Autodesk Fusion 360 part; units mm, degrees
(part 2 of 6)
  spline S17 degree 5 poles (103.1872, 58.6334) (103.1759, 58.6333) (103.1533, 58.6329) (103.1196, 58.6324) (103.0746, 58.6315) (103.0184, 58.6301) (102.9623, 58.6285) (102.9063, 58.6266) (102.8503, 58.6245) (102.7945, 58.6221) (102.7387, 58.6195) (102.683, 58.6167) (102.6274, 58.6136) (102.5718, 58.6103) (102.5164, 58.6067) (102.461, 58.6029) (102.4058, 58.5988) (102.3506, 58.5945) (102.2955, 58.5899) (102.2405, 58.585) (102.1856, 58.5799) (102.1308, 58.5746) (102.0761, 58.5689) (102.0215, 58.5631) (101.967, 58.5569) (101.9126, 58.5505) (101.8583, 58.5438) (101.8041, 58.5369) (101.75, 58.5297) (101.6961, 58.5222) (101.6422, 58.5144) (101.5884, 58.5064) (101.5348, 58.4981) (101.4813, 58.4895) (101.4279, 58.4806) (101.3746, 58.4714) (101.3215, 58.462) (101.2685, 58.4522) (101.2156, 58.4422) (101.1628, 58.4319) (101.1102, 58.4212) (101.0577, 58.4103) (101.0053, 58.3991) (100.9531, 58.3875) (100.9011, 58.3756) (100.8492, 58.3634) (100.7974, 58.3509) (100.7458, 58.3381) (100.6943, 58.325) (100.643, 58.3115) (100.5919, 58.2977) (100.541, 58.2835) (100.4902, 58.2689) (100.4397, 58.254) (100.3893, 58.2386) (100.3392, 58.223) (100.2892, 58.2069) (100.2393, 58.1906) (100.1897, 58.1739) (100.1403, 58.1567) (100.0911, 58.1391) (100.0423, 58.1209) (99.9938, 58.1022) (99.9456, 58.0828) (99.8977, 58.0629) (99.85, 58.0426) (99.8025, 58.022) (99.7552, 58.0012) (99.7081, 57.9799) (99.6615, 57.9579) (99.6156, 57.9346) (99.5797, 57.9146) (99.5534, 57.8987) (99.536, 57.8877) (99.5274, 57.882) knots -1 -1 -1 -1 -1 -1 -0.98571429 -0.97142857 -0.95714286 -0.94285714 -0.92857143 -0.91428571 -0.9 -0.88571429 -0.87142857 -0.85714286 -0.84285714 -0.82857143 -0.81428571 -0.8 -0.78571429 -0.77142857 -0.75714286 -0.74285714 -0.72857143 -0.71428571 -0.7 -0.68571429 -0.67142857 -0.65714286 -0.64285714 -0.62857143 -0.61428571 -0.6 -0.58571429 -0.57142857 -0.55714286 -0.54285714 -0.52857143 -0.51428571 -0.5 -0.48571429 -0.47142857 -0.45714286 -0.44285714 -0.42857143 -0.41428571 -0.4 -0.38571429 -0.37142857 -0.35714286 -0.34285714 -0.32857143 -0.31428571 -0.3 -0.28571429 -0.27142857 -0.25714286 -0.24285714 -0.22857143 -0.21428571 -0.2 -0.18571429 -0.17142857 -0.15714286 -0.14285714 -0.12857143 -0.11428571 -0.1 -0.08571429 -0.07142857 -0.05714286 -0.04285714 -0.02857143 -0.01428571 0 0 0 0 0 0
  line L17 (99.5274, 57.882) -> (99.1106, 57.6092)
  arc A35 (98.4247, 57.7443) -> (99.1106, 57.6092) centre (98.8368, 58.0275) ccw
  arc A36 (98.4247, 57.7443) -> (97.7326, 58.697) centre (79.882, 45) ccw
  arc A37 (97.816, 59.3911) -> (97.7326, 58.697) centre (98.1293, 59.0013) ccw
  line L18 (97.816, 59.3911) -> (98.2043, 59.7031)
  spline S18 degree 5 poles (98.2043, 59.7031) (98.2123, 59.7096) (98.2282, 59.7226) (98.2515, 59.7428) (98.2816, 59.7708) (98.3179, 59.8072) (98.3533, 59.8447) (98.388, 59.8829) (98.4225, 59.9215) (98.4567, 59.9603) (98.4907, 59.9994) (98.5245, 60.0388) (98.5578, 60.0786) (98.5906, 60.1189) (98.623, 60.1598) (98.655, 60.2011) (98.6865, 60.2428) (98.7177, 60.2848) (98.7487, 60.3272) (98.7794, 60.3698) (98.8098, 60.4127) (98.84, 60.4558) (98.8698, 60.4993) (98.8993, 60.543) (98.9286, 60.5871) (98.9575, 60.6314) (98.9862, 60.676) (99.0146, 60.7209) (99.0427, 60.766) (99.0706, 60.8114) (99.0982, 60.857) (99.1256, 60.9028) (99.1527, 60.9489) (99.1796, 60.9952) (99.2062, 61.0418) (99.2326, 61.0885) (99.2587, 61.1355) (99.2846, 61.1827) (99.3103, 61.2302) (99.3357, 61.2778) (99.3609, 61.3256) (99.3858, 61.3737) (99.4105, 61.4219) (99.435, 61.4703) (99.4593, 61.519) (99.4833, 61.5678) (99.5071, 61.6168) (99.5307, 61.666) (99.554, 61.7154) (99.5771, 61.765) (99.6, 61.8148) (99.6227, 61.8647) (99.6452, 61.9148) (99.6674, 61.9651) (99.6895, 62.0156) (99.7113, 62.0662) (99.7329, 62.117) (99.7543, 62.168) (99.7755, 62.2191) (99.7964, 62.2704) (99.8172, 62.3219) (99.8377, 62.3735) (99.858, 62.4253) (99.8782, 62.4772) (99.8981, 62.5293) (99.9178, 62.5816) (99.9373, 62.634) (99.9566, 62.6865) (99.9756, 62.7392) (99.9945, 62.7921) (100.0132, 62.8451) (100.028, 62.8876) (100.039, 62.9195) (100.0462, 62.9409) (100.0499, 62.9515) knots 0 0 0 0 0 0 0.01428571 0.02857143 0.04285714 0.05714286 0.07142857 0.08571429 0.1 0.11428571 0.12857143 0.14285714 0.15714286 0.17142857 0.18571429 0.2 0.21428571 0.22857143 0.24285714 0.25714286 0.27142857 0.28571429 0.3 0.31428571 0.32857143 0.34285714 0.35714286 0.37142857 0.38571429 0.4 0.41428571 0.42857143 0.44285714 0.45714286 0.47142857 0.48571429 0.5 0.51428571 0.52857143 0.54285714 0.55714286 0.57142857 0.58571429 0.6 0.61428571 0.62857143 0.64285714 0.65714286 0.67142857 0.68571429 0.7 0.71428571 0.72857143 0.74285714 0.75714286 0.77142857 0.78571429 0.8 0.81428571 0.82857143 0.84285714 0.85714286 0.87142857 0.88571429 0.9 0.91428571 0.92857143 0.94285714 0.95714286 0.97142857 0.98571429 1 1 1 1 1 1
  arc A38 (100.0499, 62.9515) -> (99.0645, 64.0009) centre (79.882, 45) ccw
  spline S19 degree 5 poles (99.0645, 64.0009) (99.0536, 63.9979) (99.0319, 63.992) (98.9993, 63.983) (98.9559, 63.9709) (98.9019, 63.9556) (98.8479, 63.9401) (98.7941, 63.9244) (98.7405, 63.9084) (98.687, 63.8923) (98.6336, 63.8759) (98.5803, 63.8593) (98.5272, 63.8425) (98.4743, 63.8254) (98.4215, 63.8082) (98.3688, 63.7907) (98.3163, 63.773) (98.2639, 63.7551) (98.2117, 63.7369) (98.1596, 63.7186) (98.1077, 63.7) (98.056, 63.6811) (98.0044, 63.6621) (97.953, 63.6428) (97.9017, 63.6233) (97.8506, 63.6036) (97.7997, 63.5836) (97.7489, 63.5634) (97.6983, 63.543) (97.6479, 63.5223) (97.5977, 63.5014) (97.5476, 63.4802) (97.4977, 63.4588) (97.448, 63.4372) (97.3985, 63.4153) (97.3492, 63.3932) (97.3001, 63.3708) (97.2511, 63.3482) (97.2024, 63.3253) (97.1538, 63.3022) (97.1055, 63.2788) (97.0574, 63.2552) (97.0095, 63.2313) (96.9618, 63.2071) (96.9143, 63.1826) (96.8671, 63.1579) (96.8201, 63.1329) (96.7733, 63.1077) (96.7267, 63.0822) (96.6803, 63.0564) (96.6343, 63.0303) (96.5885, 63.0038) (96.5429, 62.9771) (96.4977, 62.9501) (96.4527, 62.9227) (96.408, 62.895) (96.3636, 62.8671) (96.3194, 62.8388) (96.2755, 62.8103) (96.2319, 62.7814) (96.1886, 62.7521) (96.1458, 62.7224) (96.1035, 62.6921) (96.0617, 62.6614) (96.0202, 62.6302) (95.9791, 62.5987) (95.9382, 62.567) (95.8976, 62.535) (95.8573, 62.5027) (95.8176, 62.4697) (95.779, 62.4358) (95.7492, 62.4075) (95.7276, 62.3855) (95.7135, 62.3705) (95.7066, 62.3629) knots -1 -1 -1 -1 -1 -1 -0.98571429 -0.97142857 -0.95714286 -0.94285714 -0.92857143 -0.91428571 -0.9 -0.88571429 -0.87142857 -0.85714286 -0.84285714 -0.82857143 -0.81428571 -0.8 -0.78571429 -0.77142857 -0.75714286 -0.74285714 -0.72857143 -0.71428571 -0.7 -0.68571429 -0.67142857 -0.65714286 -0.64285714 -0.62857143 -0.61428571 -0.6 -0.58571429 -0.57142857 -0.55714286 -0.54285714 -0.52857143 -0.51428571 -0.5 -0.48571429 -0.47142857 -0.45714286 -0.44285714 -0.42857143 -0.41428571 -0.4 -0.38571429 -0.37142857 -0.35714286 -0.34285714 -0.32857143 -0.31428571 -0.3 -0.28571429 -0.27142857 -0.25714286 -0.24285714 -0.22857143 -0.21428571 -0.2 -0.18571429 -0.17142857 -0.15714286 -0.14285714 -0.12857143 -0.11428571 -0.1 -0.08571429 -0.07142857 -0.05714286 -0.04285714 -0.02857143 -0.01428571 0 0 0 0 0 0
  line L19 (95.7066, 62.3629) -> (95.3708, 61.995)
  arc A39 (94.6728, 61.9553) -> (95.3708, 61.995) centre (95.0015, 62.3321) ccw
  arc A40 (94.6728, 61.9553) -> (93.7655, 62.7059) centre (79.882, 45) ccw
  arc A41 (93.6737, 63.3989) -> (93.7655, 62.7059) centre (94.074, 63.0994) ccw
  line L20 (93.6737, 63.3989) -> (93.9722, 63.7978)
  spline S20 degree 5 poles (93.9722, 63.7978) (93.9783, 63.806) (93.9905, 63.8226) (94.008, 63.8479) (94.0302, 63.8825) (94.0563, 63.9268) (94.0812, 63.972) (94.1054, 64.0176) (94.1292, 64.0635) (94.1527, 64.1096) (94.1759, 64.1559) (94.1988, 64.2025) (94.2212, 64.2494) (94.2429, 64.2966) (94.2642, 64.3442) (94.2848, 64.3922) (94.305, 64.4404) (94.3248, 64.4889) (94.3443, 64.5376) (94.3634, 64.5865) (94.3822, 64.6356) (94.4007, 64.6849) (94.4188, 64.7344) (94.4365, 64.7841) (94.4539, 64.8341) (94.4709, 64.8842) (94.4875, 64.9346) (94.5039, 64.9851) (94.5199, 65.0358) (94.5356, 65.0867) (94.5511, 65.1377) (94.5662, 65.1889) (94.581, 65.2403) (94.5955, 65.2918) (94.6097, 65.3435) (94.6236, 65.3954) (94.6372, 65.4474) (94.6506, 65.4996) (94.6636, 65.5519) (94.6764, 65.6043) (94.6889, 65.6569) (94.7011, 65.7096) (94.713, 65.7625) (94.7247, 65.8155) (94.7361, 65.8687) (94.7472, 65.9219) (94.7581, 65.9753) (94.7687, 66.0289) (94.779, 66.0825) (94.7891, 66.1363) (94.7989, 66.1902) (94.8085, 66.2442) (94.8178, 66.2983) (94.8268, 66.3525) (94.8356, 66.4069) (94.8441, 66.4614) (94.8524, 66.516) (94.8605, 66.5706) (94.8683, 66.6254) (94.8758, 66.6803) (94.8831, 66.7354) (94.8902, 66.7905) (94.897, 66.8457) (94.9035, 66.901) (94.9099, 66.9564) (94.916, 67.0119) (94.9218, 67.0675) (94.9274, 67.1232) (94.9328, 67.179) (94.9379, 67.2349) (94.9428, 67.2909) (94.9466, 67.3357) (94.9493, 67.3694) (94.951, 67.3919) (94.9519, 67.4031) knots 0 0 0 0 0 0 0.01428571 0.02857143 0.04285714 0.05714286 0.07142857 0.08571429 0.1 0.11428571 0.12857143 0.14285714 0.15714286 0.17142857 0.18571429 0.2 0.21428571 0.22857143 0.24285714 0.25714286 0.27142857 0.28571429 0.3 0.31428571 0.32857143 0.34285714 0.35714286 0.37142857 0.38571429 0.4 0.41428571 0.42857143 0.44285714 0.45714286 0.47142857 0.48571429 0.5 0.51428571 0.52857143 0.54285714 0.55714286 0.57142857 0.58571429 0.6 0.61428571 0.62857143 0.64285714 0.65714286 0.67142857 0.68571429 0.7 0.71428571 0.72857143 0.74285714 0.75714286 0.77142857 0.78571429 0.8 0.81428571 0.82857143 0.84285714 0.85714286 0.87142857 0.88571429 0.9 0.91428571 0.92857143 0.94285714 0.95714286 0.97142857 0.98571429 1 1 1 1 1 1
  arc A42 (94.9519, 67.4031) -> (93.7365, 68.1744) centre (79.882, 45) ccw
  spline S21 degree 5 poles (93.7365, 68.1744) (93.7267, 68.1688) (93.7071, 68.1577) (93.6778, 68.1409) (93.6388, 68.1184) (93.5902, 68.0902) (93.5419, 68.0617) (93.4937, 68.0331) (93.4457, 68.0043) (93.3978, 67.9753) (93.3502, 67.9462) (93.3028, 67.9169) (93.2555, 67.8874) (93.2085, 67.8577) (93.1616, 67.8278) (93.1149, 67.7978) (93.0685, 67.7676) (93.0222, 67.7372) (92.9761, 67.7067) (92.9303, 67.6759) (92.8846, 67.645) (92.8392, 67.6139) (92.794, 67.5826) (92.749, 67.5512) (92.7042, 67.5195) (92.6596, 67.4877) (92.6152, 67.4557) (92.5711, 67.4235) (92.5271, 67.3911) (92.4834, 67.3586) (92.44, 67.3258) (92.3968, 67.2929) (92.3538, 67.2598) (92.311, 67.2264) (92.2685, 67.1929) (92.2262, 67.1592) (92.1842, 67.1254) (92.1424, 67.0913) (92.1009, 67.057) (92.0596, 67.0225) (92.0186, 66.9879) (91.9779, 66.953) (91.9375, 66.9179) (91.8973, 66.8826) (91.8574, 66.8472) (91.8178, 66.8115) (91.7784, 66.7756) (91.7394, 66.7395) (91.7006, 66.7032) (91.6622, 66.6667) (91.624, 66.6299) (91.5862, 66.5929) (91.5488, 66.5557) (91.5117, 66.5183) (91.4749, 66.4806) (91.4385, 66.4427) (91.4024, 66.4045) (91.3667, 66.3662) (91.3312, 66.3276) (91.2961, 66.2888) (91.2616, 66.2497) (91.2275, 66.2102) (91.194, 66.1704) (91.1612, 66.1302) (91.1288, 66.0897) (91.0968, 66.049) (91.0651, 66.0081) (91.0336, 65.967) (91.0027, 65.9257) (90.9724, 65.8839) (90.9434, 65.8414) (90.9216, 65.8066) (90.9061, 65.78) (90.8963, 65.7619) (90.8915, 65.7529) knots -1 -1 -1 -1 -1 -1 -0.98571429 -0.97142857 -0.95714286 -0.94285714 -0.92857143 -0.91428571 -0.9 -0.88571429 -0.87142857 -0.85714286 -0.84285714 -0.82857143 -0.81428571 -0.8 -0.78571429 -0.77142857 -0.75714286 -0.74285714 -0.72857143 -0.71428571 -0.7 -0.68571429 -0.67142857 -0.65714286 -0.64285714 -0.62857143 -0.61428571 -0.6 -0.58571429 -0.57142857 -0.55714286 -0.54285714 -0.52857143 -0.51428571 -0.5 -0.48571429 -0.47142857 -0.45714286 -0.44285714 -0.42857143 -0.41428571 -0.4 -0.38571429 -0.37142857 -0.35714286 -0.34285714 -0.32857143 -0.31428571 -0.3 -0.28571429 -0.27142857 -0.25714286 -0.24285714 -0.22857143 -0.21428571 -0.2 -0.18571429 -0.17142857 -0.15714286 -0.14285714 -0.12857143 -0.11428571 -0.1 -0.08571429 -0.07142857 -0.05714286 -0.04285714 -0.02857143 -0.01428571 0 0 0 0 0 0
  line L21 (90.8915, 65.7529) -> (90.6577, 65.313)
  arc A43 (89.9915, 65.101) -> (90.6577, 65.313) centre (90.2161, 65.5476) ccw
  arc A44 (89.9915, 65.101) -> (88.926, 65.6023) centre (79.882, 45) ccw
  arc A45 (88.6648, 66.2508) -> (88.926, 65.6023) centre (89.127, 66.0601) ccw
  line L22 (88.6648, 66.2508) -> (88.8547, 66.7113)
  spline S22 degree 5 poles (88.8547, 66.7113) (88.8586, 66.7208) (88.8662, 66.7399) (88.8769, 66.7688) (88.8898, 66.8078) (88.9041, 66.8572) (88.917, 66.9071) (88.929, 66.9573) (88.9407, 67.0077) (88.952, 67.0582) (88.963, 67.1089) (88.9735, 67.1596) (88.9835, 67.2106) (88.9929, 67.2618) (89.0016, 67.3132) (89.0097, 67.3647) (89.0173, 67.4165) (89.0244, 67.4684) (89.0311, 67.5204) (89.0375, 67.5725) (89.0435, 67.6247) (89.0491, 67.6771) (89.0543, 67.7295) (89.0591, 67.7821) (89.0635, 67.8348) (89.0675, 67.8876) (89.0711, 67.9405) (89.0744, 67.9935) (89.0773, 68.0466) (89.0799, 68.0998) (89.0822, 68.1531) (89.0841, 68.2064) (89.0856, 68.2599) (89.0869, 68.3134) (89.0878, 68.367) (89.0884, 68.4207) (89.0886, 68.4745) (89.0886, 68.5283) (89.0882, 68.5822) (89.0875, 68.6362) (89.0865, 68.6903) (89.0852, 68.7444) (89.0837, 68.7985) (89.0818, 68.8528) (89.0796, 68.9071) (89.0771, 68.9615) (89.0744, 69.0159) (89.0713, 69.0704) (89.068, 69.1249) (89.0644, 69.1795) (89.0605, 69.2341) (89.0563, 69.2888) (89.0518, 69.3435) (89.0471, 69.3983) (89.0421, 69.4532) (89.0368, 69.5081) (89.0313, 69.563) (89.0255, 69.618) (89.0194, 69.673) (89.0131, 69.728) (89.0064, 69.7831) (88.9996, 69.8382) (88.9924, 69.8934) (88.9851, 69.9486) (88.9774, 70.0039) (88.9695, 70.0592) (88.9613, 70.1145) (88.9529, 70.1698) (88.9443, 70.2252) (88.9353, 70.2806) (88.9262, 70.336) (88.9186, 70.3804) (88.9129, 70.4137) (88.909, 70.4359) (88.907, 70.447) knots 0 0 0 0 0 0 0.01428571 0.02857143 0.04285714 0.05714286 0.07142857 0.08571429 0.1 0.11428571 0.12857143 0.14285714 0.15714286 0.17142857 0.18571429 0.2 0.21428571 0.22857143 0.24285714 0.25714286 0.27142857 0.28571429 0.3 0.31428571 0.32857143 0.34285714 0.35714286 0.37142857 0.38571429 0.4 0.41428571 0.42857143 0.44285714 0.45714286 0.47142857 0.48571429 0.5 0.51428571 0.52857143 0.54285714 0.55714286 0.57142857 0.58571429 0.6 0.61428571 0.62857143 0.64285714 0.65714286 0.67142857 0.68571429 0.7 0.71428571 0.72857143 0.74285714 0.75714286 0.77142857 0.78571429 0.8 0.81428571 0.82857143 0.84285714 0.85714286 0.87142857 0.88571429 0.9 0.91428571 0.92857143 0.94285714 0.95714286 0.97142857 0.98571429 1 1 1 1 1 1
  arc A46 (88.907, 70.447) -> (87.538, 70.8918) centre (79.882, 45) ccw
  spline S23 degree 5 poles (87.538, 70.8918) (87.5299, 70.884) (87.5137, 70.8683) (87.4895, 70.8448) (87.4573, 70.8133) (87.4173, 70.7738) (87.3775, 70.7343) (87.3379, 70.6945) (87.2986, 70.6547) (87.2595, 70.6148) (87.2206, 70.5747) (87.1819, 70.5345) (87.1435, 70.4942) (87.1053, 70.4537) (87.0673, 70.4132) (87.0296, 70.3725) (86.9921, 70.3317) (86.9549, 70.2907) (86.9179, 70.2497) (86.8811, 70.2085) (86.8446, 70.1672) (86.8083, 70.1258) (86.7722, 70.0842) (86.7365, 70.0426) (86.7009, 70.0008) (86.6657, 69.9589) (86.6307, 69.9168) (86.5959, 69.8747) (86.5614, 69.8324) (86.5272, 69.79) (86.4932, 69.7475) (86.4596, 69.7048) (86.4262, 69.662) (86.393, 69.6191) (86.3602, 69.5761) (86.3276, 69.533) (86.2954, 69.4897) (86.2634, 69.4463) (86.2317, 69.4028) (86.2003, 69.3591) (86.1692, 69.3153) (86.1384, 69.2714) (86.108, 69.2274) (86.0778, 69.1832) (86.048, 69.1389) (86.0185, 69.0945) (85.9893, 69.05) (85.9605, 69.0053) (85.932, 68.9605) (85.9038, 68.9156) (85.876, 68.8705) (85.8486, 68.8253) (85.8216, 68.7799) (85.7949, 68.7344) (85.7687, 68.6888) (85.7429, 68.643) (85.7174, 68.5971) (85.6923, 68.551) (85.6675, 68.5049) (85.6432, 68.4586) (85.6195, 68.4121) (85.5963, 68.3654) (85.5738, 68.3185) (85.5519, 68.2714) (85.5306, 68.2241) (85.5098, 68.1767) (85.4892, 68.1292) (85.469, 68.0816) (85.4493, 68.0339) (85.4304, 67.9859) (85.4129, 67.9375) (85.4004, 67.8984) (85.392, 67.8687) (85.387, 67.8488) (85.3845, 67.8388) knots -1 -1 -1 -1 -1 -1 -0.98571429 -0.97142857 -0.95714286 -0.94285714 -0.92857143 -0.91428571 -0.9 -0.88571429 -0.87142857 -0.85714286 -0.84285714 -0.82857143 -0.81428571 -0.8 -0.78571429 -0.77142857 -0.75714286 -0.74285714 -0.72857143 -0.71428571 -0.7 -0.68571429 -0.67142857 -0.65714286 -0.64285714 -0.62857143 -0.61428571 -0.6 -0.58571429 -0.57142857 -0.55714286 -0.54285714 -0.52857143 -0.51428571 -0.5 -0.48571429 -0.47142857 -0.45714286 -0.44285714 -0.42857143 -0.41428571 -0.4 -0.38571429 -0.37142857 -0.35714286 -0.34285714 -0.32857143 -0.31428571 -0.3 -0.28571429 -0.27142857 -0.25714286 -0.24285714 -0.22857143 -0.21428571 -0.2 -0.18571429 -0.17142857 -0.15714286 -0.14285714 -0.12857143 -0.11428571 -0.1 -0.08571429 -0.07142857 -0.05714286 -0.04285714 -0.02857143 -0.01428571 0 0 0 0 0 0
  line L23 (85.3845, 67.8388) -> (85.2675, 67.3546)
  arc A47 (84.675, 66.9836) -> (85.2675, 67.3546) centre (84.7815, 67.4721) ccw
  arc A48 (84.675, 66.9836) -> (83.5183, 67.2042) centre (79.882, 45) ccw
  arc A49 (83.104, 67.7673) -> (83.5183, 67.2042) centre (83.5991, 67.6976) ccw
  line L24 (83.104, 67.7673) -> (83.1734, 68.2606)
  spline S24 degree 5 poles (83.1734, 68.2606) (83.1749, 68.2708) (83.1775, 68.2912) (83.1806, 68.3218) (83.1834, 68.3628) (83.1849, 68.4142) (83.185, 68.4658) (83.1842, 68.5174) (83.183, 68.5691) (83.1814, 68.6209) (83.1794, 68.6726) (83.177, 68.7244) (83.174, 68.7763) (83.1704, 68.8282) (83.166, 68.8801) (83.161, 68.9321) (83.1555, 68.9841) (83.1495, 69.0361) (83.1431, 69.0882) (83.1363, 69.1402) (83.1291, 69.1923) (83.1215, 69.2444) (83.1135, 69.2965) (83.1051, 69.3486) (83.0963, 69.4008) (83.087, 69.4529) (83.0774, 69.505) (83.0674, 69.5572) (83.057, 69.6094) (83.0462, 69.6615) (83.0352, 69.7137) (83.0238, 69.7658) (83.012, 69.818) (82.9999, 69.8701) (82.9874, 69.9223) (82.9746, 69.9744) (82.9615, 70.0266) (82.9481, 70.0787) (82.9343, 70.1308) (82.9202, 70.1829) (82.9058, 70.2351) (82.8911, 70.2871) (82.8761, 70.3392) (82.8608, 70.3913) (82.8452, 70.4434) (82.8293, 70.4954) (82.8131, 70.5474) (82.7966, 70.5994) (82.7798, 70.6514) (82.7627, 70.7034) (82.7453, 70.7553) (82.7277, 70.8073) (82.7098, 70.8592) (82.6916, 70.9111) (82.6731, 70.963) (82.6543, 71.0148) (82.6353, 71.0666) (82.616, 71.1184) (82.5964, 71.1702) (82.5766, 71.2219) (82.5565, 71.2737) (82.5361, 71.3254) (82.5155, 71.377) (82.4946, 71.4287) (82.4734, 71.4803) (82.452, 71.5318) (82.4304, 71.5834) (82.4085, 71.6349) (82.3863, 71.6864) (82.3639, 71.7378) (82.3412, 71.7892) (82.3229, 71.8303) (82.309, 71.8612) (82.2997, 71.8817) (82.2951, 71.892) knots 0 0 0 0 0 0 0.01428571 0.02857143 0.04285714 0.05714286 0.07142857 0.08571429 0.1 0.11428571 0.12857143 0.14285714 0.15714286 0.17142857 0.18571429 0.2 0.21428571 0.22857143 0.24285714 0.25714286 0.27142857 0.28571429 0.3 0.31428571 0.32857143 0.34285714 0.35714286 0.37142857 0.38571429 0.4 0.41428571 0.42857143 0.44285714 0.45714286 0.47142857 0.48571429 0.5 0.51428571 0.52857143 0.54285714 0.55714286 0.57142857 0.58571429 0.6 0.61428571 0.62857143 0.64285714 0.65714286 0.67142857 0.68571429 0.7 0.71428571 0.72857143 0.74285714 0.75714286 0.77142857 0.78571429 0.8 0.81428571 0.82857143 0.84285714 0.85714286 0.87142857 0.88571429 0.9 0.91428571 0.92857143 0.94285714 0.95714286 0.97142857 0.98571429 1 1 1 1 1 1
  arc A50 (82.2951, 71.892) -> (80.8584, 71.9823) centre (79.882, 45) ccw
  spline S25 degree 5 poles (80.8584, 71.9823) (80.8525, 71.9727) (80.8407, 71.9535) (80.8231, 71.9247) (80.7998, 71.8862) (80.7709, 71.838) (80.7422, 71.7898) (80.7137, 71.7415) (80.6855, 71.6932) (80.6576, 71.6447) (80.6299, 71.5962) (80.6024, 71.5477) (80.5752, 71.4991) (80.5483, 71.4504) (80.5216, 71.4017) (80.4952, 71.3529) (80.469, 71.304) (80.4431, 71.2551) (80.4175, 71.2062) (80.3921, 71.1571) (80.367, 71.108) (80.3421, 71.0589) (80.3176, 71.0097) (80.2933, 70.9604) (80.2693, 70.9111) (80.2455, 70.8618) (80.2221, 70.8123) (80.1989, 70.7629) (80.176, 70.7133) (80.1534, 70.6637) (80.1311, 70.6141) (80.1091, 70.5644) (80.0874, 70.5147) (80.066, 70.4649) (80.0448, 70.4151) (80.024, 70.3652) (80.0035, 70.3152) (79.9833, 70.2652) (79.9635, 70.2152) (79.9439, 70.1651) (79.9247, 70.115) (79.9058, 70.0648) (79.8872, 70.0146) (79.869, 69.9643) (79.8512, 69.914) (79.8336, 69.8636) (79.8165, 69.8132) (79.7996, 69.7628) (79.7831, 69.7123) (79.767, 69.6618) (79.7513, 69.6112) (79.736, 69.5606) (79.7211, 69.5099) (79.7067, 69.4592) (79.6926, 69.4085) (79.679, 69.3577) (79.6657, 69.3069) (79.6528, 69.2561) (79.6404, 69.2052) (79.6283, 69.1543) (79.6169, 69.1034) (79.606, 69.0524) (79.5959, 69.0014) (79.5864, 68.9503) (79.5776, 68.8992) (79.5692, 68.8481) (79.5611, 68.797) (79.5533, 68.7459) (79.5461, 68.6947) (79.5397, 68.6436) (79.5348, 68.5924) (79.5324, 68.5513) (79.5317, 68.5205) (79.5317, 68.5) (79.5319, 68.4897) knots -1 -1 -1 -1 -1 -1 -0.98571429 -0.97142857 -0.95714286 -0.94285714 -0.92857143 -0.91428571 -0.9 -0.88571429 -0.87142857 -0.85714286 -0.84285714 -0.82857143 -0.81428571 -0.8 -0.78571429 -0.77142857 -0.75714286 -0.74285714 -0.72857143 -0.71428571 -0.7 -0.68571429 -0.67142857 -0.65714286 -0.64285714 -0.62857143 -0.61428571 -0.6 -0.58571429 -0.57142857 -0.55714286 -0.54285714 -0.52857143 -0.51428571 -0.5 -0.48571429 -0.47142857 -0.45714286 -0.44285714 -0.42857143 -0.41428571 -0.4 -0.38571429 -0.37142857 -0.35714286 -0.34285714 -0.32857143 -0.31428571 -0.3 -0.28571429 -0.27142857 -0.25714286 -0.24285714 -0.22857143 -0.21428571 -0.2 -0.18571429 -0.17142857 -0.15714286 -0.14285714 -0.12857143 -0.11428571 -0.1 -0.08571429 -0.07142857 -0.05714286 -0.04285714 -0.02857143 -0.01428571 0 0 0 0 0 0
  line L25 (79.5319, 68.4897) -> (79.5389, 67.9916)
  arc A51 (79.0573, 67.4849) -> (79.5389, 67.9916) centre (79.039, 67.9845) ccw
  arc A52 (79.0573, 67.4849) -> (77.8821, 67.4109) centre (79.882, 45) ccw
  arc A53 (77.3408, 67.8533) -> (77.8821, 67.4109) centre (77.8377, 67.909) ccw
  line L26 (77.3408, 67.8533) -> (77.2853, 68.3484)
  spline S26 degree 5 poles (77.2853, 68.3484) (77.2842, 68.3586) (77.2817, 68.379) (77.2771, 68.4095) (77.2696, 68.4499) (77.2583, 68.5) (77.2456, 68.55) (77.232, 68.5998) (77.2179, 68.6496) (77.2034, 68.6993) (77.1887, 68.7489) (77.1735, 68.7985) (77.1577, 68.848) (77.1413, 68.8973) (77.1241, 68.9466) (77.1064, 68.9957) (77.0881, 69.0447) (77.0693, 69.0936) (77.0501, 69.1424) (77.0306, 69.1911) (77.0107, 69.2398) (76.9904, 69.2884) (76.9697, 69.3368) (76.9486, 69.3852) (76.9271, 69.4335) (76.9051, 69.4817) (76.8828, 69.5298) (76.8602, 69.5779) (76.8371, 69.6258) (76.8138, 69.6736) (76.7901, 69.7214) (76.766, 69.7691) (76.7417, 69.8167) (76.717, 69.8642) (76.6919, 69.9116) (76.6666, 69.9589) (76.6409, 70.0062) (76.6149, 70.0533) (76.5886, 70.1004) (76.562, 70.1474) (76.5351, 70.1942) (76.5079, 70.241) (76.4804, 70.2878) (76.4527, 70.3344) (76.4246, 70.3809) (76.3962, 70.4274) (76.3676, 70.4737) (76.3387, 70.52) (76.3095, 70.5662) (76.28, 70.6123) (76.2503, 70.6583) (76.2203, 70.7042) (76.19, 70.75) (76.1595, 70.7957) (76.1287, 70.8414) (76.0976, 70.8869) (76.0663, 70.9324) (76.0347, 70.9778) (76.0029, 71.0231) (75.9708, 71.0682) (75.9385, 71.1133) (75.9059, 71.1583) (75.8731, 71.2033) (75.84, 71.2481) (75.8067, 71.2928) (75.7731, 71.3374) (75.7393, 71.382) (75.7053, 71.4264) (75.671, 71.4708) (75.6365, 71.515) (75.6017, 71.5592) (75.5738, 71.5944) (75.5527, 71.6208) (75.5386, 71.6384) (75.5315, 71.6472) knots 0 0 0 0 0 0 0.01428571 0.02857143 0.04285714 0.05714286 0.07142857 0.08571429 0.1 0.11428571 0.12857143 0.14285714 0.15714286 0.17142857 0.18571429 0.2 0.21428571 0.22857143 0.24285714 0.25714286 0.27142857 0.28571429 0.3 0.31428571 0.32857143 0.34285714 0.35714286 0.37142857 0.38571429 0.4 0.41428571 0.42857143 0.44285714 0.45714286 0.47142857 0.48571429 0.5 0.51428571 0.52857143 0.54285714 0.55714286 0.57142857 0.58571429 0.6 0.61428571 0.62857143 0.64285714 0.65714286 0.67142857 0.68571429 0.7 0.71428571 0.72857143 0.74285714 0.75714286 0.77142857 0.78571429 0.8 0.81428571 0.82857143 0.84285714 0.85714286 0.87142857 0.88571429 0.9 0.91428571 0.92857143 0.94285714 0.95714286 0.97142857 0.98571429 1 1 1 1 1 1
  arc A54 (75.5315, 71.6472) -> (74.1175, 71.3775) centre (79.882, 45) ccw
  spline S27 degree 5 poles (74.1175, 71.3775) (74.1142, 71.3667) (74.1076, 71.3452) (74.0977, 71.3129) (74.0846, 71.2698) (74.0686, 71.2159) (74.0528, 71.1621) (74.0372, 71.1082) (74.022, 71.0544) (74.0069, 71.0005) (73.9922, 70.9467) (73.9776, 70.8928) (73.9634, 70.839) (73.9494, 70.7851) (73.9357, 70.7313) (73.9222, 70.6775) (73.909, 70.6236) (73.8961, 70.5698) (73.8834, 70.516) (73.8711, 70.4622) (73.8589, 70.4084) (73.8471, 70.3546) (73.8355, 70.3009) (73.8243, 70.2471) (73.8133, 70.1934) (73.8026, 70.1397) (73.7921, 70.086) (73.782, 70.0323) (73.7721, 69.9786) (73.7626, 69.925) (73.7533, 69.8713) (73.7443, 69.8177) (73.7357, 69.7642) (73.7273, 69.7106) (73.7193, 69.6571) (73.7115, 69.6036) (73.7041, 69.5501) (73.697, 69.4967) (73.6901, 69.4433) (73.6837, 69.3899) (73.6775, 69.3366) (73.6717, 69.2833) (73.6662, 69.23) (73.6611, 69.1768) (73.6563, 69.1236) (73.6518, 69.0705) (73.6477, 69.0174) (73.644, 68.9643) (73.6406, 68.9113) (73.6375, 68.8584) (73.6349, 68.8055) (73.6326, 68.7527) (73.6308, 68.6999) (73.6294, 68.6472) (73.6284, 68.5946) (73.6278, 68.542) (73.6276, 68.4895) (73.6278, 68.4371) (73.6283, 68.3847) (73.6294, 68.3324) (73.6309, 68.2802) (73.6331, 68.2281) (73.636, 68.1762) (73.6395, 68.1244) (73.6436, 68.0727) (73.6482, 68.0211) (73.6531, 67.9696) (73.6583, 67.9181) (73.664, 67.8668) (73.6705, 67.8156) (73.6785, 67.7648) (73.6864, 67.7245) (73.6934, 67.6945) (73.6985, 67.6746) (73.7012, 67.6647) knots -1 -1 -1 -1 -1 -1 -0.98571429 -0.97142857 -0.95714286 -0.94285714 -0.92857143 -0.91428571 -0.9 -0.88571429 -0.87142857 -0.85714286 -0.84285714 -0.82857143 -0.81428571 -0.8 -0.78571429 -0.77142857 -0.75714286 -0.74285714 -0.72857143 -0.71428571 -0.7 -0.68571429 -0.67142857 -0.65714286 -0.64285714 -0.62857143 -0.61428571 -0.6 -0.58571429 -0.57142857 -0.55714286 -0.54285714 -0.52857143 -0.51428571 -0.5 -0.48571429 -0.47142857 -0.45714286 -0.44285714 -0.42857143 -0.41428571 -0.4 -0.38571429 -0.37142857 -0.35714286 -0.34285714 -0.32857143 -0.31428571 -0.3 -0.28571429 -0.27142857 -0.25714286 -0.24285714 -0.22857143 -0.21428571 -0.2 -0.18571429 -0.17142857 -0.15714286 -0.14285714 -0.12857143 -0.11428571 -0.1 -0.08571429 -0.07142857 -0.05714286 -0.04285714 -0.02857143 -0.01428571 0 0 0 0 0 0
  line L27 (73.7012, 67.6647) -> (73.8319, 67.184)
  arc A55 (73.4915, 66.5734) -> (73.8319, 67.184) centre (73.3494, 67.0528) ccw
  arc A56 (73.4915, 66.5734) -> (72.3716, 66.2095) centre (79.882, 45) ccw
  arc A57 (71.7372, 66.5034) -> (72.3716, 66.2095) centre (72.2047, 66.6808) ccw
  line L28 (71.7372, 66.5034) -> (71.5604, 66.9691)
  spline S28 degree 5 poles (71.5604, 66.9691) (71.5568, 66.9787) (71.5492, 66.9978) (71.5372, 67.0262) (71.5199, 67.0635) (71.4965, 67.1092) (71.4718, 67.1545) (71.4462, 67.1993) (71.4202, 67.244) (71.3938, 67.2886) (71.3672, 67.333) (71.3401, 67.3773) (71.3125, 67.4213) (71.2843, 67.465) (71.2555, 67.5084) (71.2261, 67.5515) (71.1962, 67.5944) (71.1658, 67.6371) (71.1351, 67.6796) (71.1041, 67.722) (71.0727, 67.7642) (71.041, 67.8062) (71.0089, 67.848) (70.9764, 67.8896) (70.9435, 67.931) (70.9103, 67.9723) (70.8767, 68.0133) (70.8428, 68.0542) (70.8086, 68.0949) (70.7741, 68.1354) (70.7392, 68.1758) (70.7041, 68.216) (70.6687, 68.256) (70.6329, 68.2959) (70.5969, 68.3356) (70.5606, 68.3751) (70.5239, 68.4145) (70.487, 68.4537) (70.4499, 68.4928) (70.4124, 68.5317) (70.3747, 68.5704) (70.3367, 68.6089) (70.2985, 68.6474) (70.26, 68.6856) (70.2212, 68.7237) (70.1822, 68.7616) (70.143, 68.7994) (70.1034, 68.837) (70.0637, 68.8745) (70.0237, 68.9118) (69.9834, 68.949) (69.943, 68.986) (69.9022, 69.0229) (69.8613, 69.0596) (69.8201, 69.0961) (69.7787, 69.1325) (69.737, 69.1688) (69.6952, 69.2048) (69.6531, 69.2408) (69.6108, 69.2766) (69.5682, 69.3122) (69.5255, 69.3477) (69.4825, 69.383) (69.4393, 69.4182) (69.3959, 69.4533) (69.3523, 69.4881) (69.3085, 69.5229) (69.2645, 69.5575) (69.2203, 69.5919) (69.1759, 69.6262) (69.1312, 69.6603) (69.0954, 69.6875) (69.0684, 69.7078) (69.0503, 69.7213) (69.0413, 69.7281) knots 0 0 0 0 0 0 0.01428571 0.02857143 0.04285714 0.05714286 0.07142857 0.08571429 0.1 0.11428571 0.12857143 0.14285714 0.15714286 0.17142857 0.18571429 0.2 0.21428571 0.22857143 0.24285714 0.25714286 0.27142857 0.28571429 0.3 0.31428571 0.32857143 0.34285714 0.35714286 0.37142857 0.38571429 0.4 0.41428571 0.42857143 0.44285714 0.45714286 0.47142857 0.48571429 0.5 0.51428571 0.52857143 0.54285714 0.55714286 0.57142857 0.58571429 0.6 0.61428571 0.62857143 0.64285714 0.65714286 0.67142857 0.68571429 0.7 0.71428571 0.72857143 0.74285714 0.75714286 0.77142857 0.78571429 0.8 0.81428571 0.82857143 0.84285714 0.85714286 0.87142857 0.88571429 0.9 0.91428571 0.92857143 0.94285714 0.95714286 0.97142857 0.98571429 1 1 1 1 1 1
  arc A58 (69.0413, 69.7281) -> (67.7388, 69.1152) centre (79.882, 45) ccw
  spline S29 degree 5 poles (67.7388, 69.1152) (67.7383, 69.1039) (67.7372, 69.0814) (67.7356, 69.0477) (67.7337, 69.0027) (67.7316, 68.9466) (67.7297, 68.8905) (67.728, 68.8344) (67.7266, 68.7785) (67.7254, 68.7226) (67.7245, 68.6668) (67.7239, 68.611) (67.7235, 68.5553) (67.7233, 68.4997) (67.7234, 68.4441) (67.7237, 68.3886) (67.7243, 68.3332) (67.7252, 68.2779) (67.7263, 68.2226) (67.7277, 68.1674) (67.7294, 68.1123) (67.7313, 68.0573) (67.7334, 68.0023) (67.7359, 67.9474) (67.7386, 67.8927) (67.7416, 67.838) (67.7448, 67.7833) (67.7484, 67.7288) (67.7522, 67.6744) (67.7562, 67.6201) (67.7606, 67.5658) (67.7652, 67.5117) (67.7702, 67.4576) (67.7754, 67.4037) (67.7809, 67.3498) (67.7867, 67.2961) (67.7928, 67.2424) (67.7992, 67.1889) (67.8059, 67.1355) (67.8129, 67.0822) (67.8202, 67.029) (67.8278, 66.9759) (67.8357, 66.923) (67.844, 66.8701) (67.8526, 66.8174) (67.8615, 66.7649) (67.8707, 66.7124) (67.8803, 66.6601) (67.8901, 66.6079) (67.9004, 66.5559) (67.9109, 66.504) (67.9219, 66.4523) (67.9333, 66.4007) (67.945, 66.3493) (67.9572, 66.2981) (67.9697, 66.247) (67.9825, 66.1961) (67.9957, 66.1454) (68.0093, 66.0948) (68.0233, 66.0444) (68.0378, 65.9942) (68.0528, 65.9443) (68.0685, 65.8947) (68.0848, 65.8454) (68.1017, 65.7964) (68.1189, 65.7475) (68.1365, 65.6989) (68.1543, 65.6503) (68.1726, 65.602) (68.1917, 65.5541) (68.212, 65.5069) (68.2297, 65.4698) (68.2439, 65.4424) (68.2539, 65.4245) (68.2589, 65.4155) knots -1 -1 -1 -1 -1 -1 -0.98571429 -0.97142857 -0.95714286 -0.94285714 -0.92857143 -0.91428571 -0.9 -0.88571429 -0.87142857 -0.85714286 -0.84285714 -0.82857143 -0.81428571 -0.8 -0.78571429 -0.77142857 -0.75714286 -0.74285714 -0.72857143 -0.71428571 -0.7 -0.68571429 -0.67142857 -0.65714286 -0.64285714 -0.62857143 -0.61428571 -0.6 -0.58571429 -0.57142857 -0.55714286 -0.54285714 -0.52857143 -0.51428571 -0.5 -0.48571429 -0.47142857 -0.45714286 -0.44285714 -0.42857143 -0.41428571 -0.4 -0.38571429 -0.37142857 -0.35714286 -0.34285714 -0.32857143 -0.31428571 -0.3 -0.28571429 -0.27142857 -0.25714286 -0.24285714 -0.22857143 -0.21428571 -0.2 -0.18571429 -0.17142857 -0.15714286 -0.14285714 -0.12857143 -0.11428571 -0.1 -0.08571429 -0.07142857 -0.05714286 -0.04285714 -0.02857143 -0.01428571 0 0 0 0 0 0
  line L29 (68.2589, 65.4155) -> (68.5051, 64.9824)
  arc A59 (68.3271, 64.3063) -> (68.5051, 64.9824) centre (68.0704, 64.7354) ccw
  arc A60 (68.3271, 64.3063) -> (67.3329, 63.6754) centre (79.882, 45) ccw
  arc A61 (66.6454, 63.8023) -> (67.3329, 63.6754) centre (67.0541, 64.0904) ccw
  line L30 (66.6454, 63.8023) -> (66.3584, 64.2094)
  spline S30 degree 5 poles (66.3584, 64.2094) (66.3524, 64.2178) (66.3404, 64.2344) (66.3217, 64.2589) (66.2957, 64.2907) (66.2616, 64.3293) (66.2264, 64.3669) (66.1905, 64.404) (66.1541, 64.4408) (66.1175, 64.4774) (66.0807, 64.5138) (66.0435, 64.55) (66.0058, 64.5857) (65.9676, 64.621) (65.9289, 64.6559) (65.8897, 64.6904) (65.85, 64.7245) (65.81, 64.7583) (65.7697, 64.7919) (65.7291, 64.8252) (65.6883, 64.8582) (65.6471, 64.891) (65.6056, 64.9235) (65.5638, 64.9558) (65.5216, 64.9877) (65.4792, 65.0194) (65.4365, 65.0508) (65.3935, 65.0819) (65.3502, 65.1129) (65.3067, 65.1435) (65.2629, 65.174) (65.2189, 65.2042) (65.1746, 65.2341) (65.1301, 65.2639) (65.0853, 65.2934) (65.0403, 65.3226) (64.995, 65.3516) (64.9495, 65.3804) (64.9038, 65.409) (64.8579, 65.4374) (64.8117, 65.4655) (64.7653, 65.4934) (64.7187, 65.5211) (64.6719, 65.5486) (64.6249, 65.5758) (64.5777, 65.6029) (64.5303, 65.6297) (64.4826, 65.6563) (64.4348, 65.6827) (64.3868, 65.7089) (64.3385, 65.7349) (64.2901, 65.7607) (64.2415, 65.7863) (64.1927, 65.8116) (64.1437, 65.8368) (64.0946, 65.8617) (64.0452, 65.8865) (63.9957, 65.911) (63.946, 65.9354) (63.8961, 65.9595) (63.8461, 65.9835) (63.7958, 66.0072) (63.7454, 66.0308) (63.6948, 66.0541) (63.6441, 66.0772) (63.5932, 66.1002) (63.5421, 66.1229) (63.4909, 66.1455) (63.4395, 66.1678) (63.3879, 66.19) (63.3362, 66.212) (63.2947, 66.2294) (63.2635, 66.2423) (63.2427, 66.2509) (63.2322, 66.2552) knots 0 0 0 0 0 0 0.01428571 0.02857143 0.04285714 0.05714286 0.07142857 0.08571429 0.1 0.11428571 0.12857143 0.14285714 0.15714286 0.17142857 0.18571429 0.2 0.21428571 0.22857143 0.24285714 0.25714286 0.27142857 0.28571429 0.3 0.31428571 0.32857143 0.34285714 0.35714286 0.37142857 0.38571429 0.4 0.41428571 0.42857143 0.44285714 0.45714286 0.47142857 0.48571429 0.5 0.51428571 0.52857143 0.54285714 0.55714286 0.57142857 0.58571429 0.6 0.61428571 0.62857143 0.64285714 0.65714286 0.67142857 0.68571429 0.7 0.71428571 0.72857143 0.74285714 0.75714286 0.77142857 0.78571429 0.8 0.81428571 0.82857143 0.84285714 0.85714286 0.87142857 0.88571429 0.9 0.91428571 0.92857143 0.94285714 0.95714286 0.97142857 0.98571429 1 1 1 1 1 1
  arc A62 (63.2322, 66.2552) -> (62.1231, 65.3377) centre (79.882, 45) ccw
  spline S31 degree 5 poles (62.1231, 65.3377) (62.1254, 65.3266) (62.1299, 65.3046) (62.1368, 65.2715) (62.1462, 65.2275) (62.158, 65.1725) (62.1701, 65.1177) (62.1825, 65.0631) (62.195, 65.0085) (62.2078, 64.9541) (62.2208, 64.8998) (62.234, 64.8456) (62.2475, 64.7915) (62.2612, 64.7376) (62.2751, 64.6838) (62.2892, 64.6302) (62.3036, 64.5766) (62.3182, 64.5233) (62.333, 64.47) (62.3481, 64.4169) (62.3634, 64.3639) (62.3789, 64.3111) (62.3947, 64.2584) (62.4107, 64.2059) (62.4269, 64.1535) (62.4434, 64.1013) (62.4601, 64.0492) (62.4771, 63.9972) (62.4943, 63.9455) (62.5118, 63.8938) (62.5295, 63.8424) (62.5475, 63.7911) (62.5657, 63.74) (62.5842, 63.689) (62.6029, 63.6382) (62.6219, 63.5876) (62.6411, 63.5372) (62.6606, 63.4869) (62.6804, 63.4368) (62.7004, 63.387) (62.7207, 63.3372) (62.7413, 63.2877) (62.7622, 63.2384) (62.7833, 63.1893) (62.8047, 63.1404) (62.8264, 63.0917) (62.8484, 63.0432) (62.8707, 62.9949) (62.8932, 62.9468) (62.9161, 62.899) (62.9392, 62.8513) (62.9627, 62.804) (62.9865, 62.7568) (63.0107, 62.71) (63.0352, 62.6634) (63.06, 62.6171) (63.0851, 62.5709) (63.1105, 62.5251) (63.1362, 62.4794) (63.1623, 62.4341) (63.1888, 62.3891) (63.2158, 62.3445) (63.2434, 62.3004) (63.2714, 62.2567) (63.2999, 62.2134) (63.3288, 62.1704) (63.3579, 62.1276) (63.3873, 62.085) (63.417, 62.0427) (63.4473, 62.0011) (63.4788, 61.9604) (63.5052, 61.9289) (63.5257, 61.9059) (63.5398, 61.891) (63.547, 61.8836) knots -1 -1 -1 -1 -1 -1 -0.98571429 -0.97142857 -0.95714286 -0.94285714 -0.92857143 -0.91428571 -0.9 -0.88571429 -0.87142857 -0.85714286 -0.84285714 -0.82857143 -0.81428571 -0.8 -0.78571429 -0.77142857 -0.75714286 -0.74285714 -0.72857143 -0.71428571 -0.7 -0.68571429 -0.67142857 -0.65714286 -0.64285714 -0.62857143 -0.61428571 -0.6 -0.58571429 -0.57142857 -0.55714286 -0.54285714 -0.52857143 -0.51428571 -0.5 -0.48571429 -0.47142857 -0.45714286 -0.44285714 -0.42857143 -0.41428571 -0.4 -0.38571429 -0.37142857 -0.35714286 -0.34285714 -0.32857143 -0.31428571 -0.3 -0.28571429 -0.27142857 -0.25714286 -0.24285714 -0.22857143 -0.21428571 -0.2 -0.18571429 -0.17142857 -0.15714286 -0.14285714 -0.12857143 -0.11428571 -0.1 -0.08571429 -0.07142857 -0.05714286 -0.04285714 -0.02857143 -0.01428571 0 0 0 0 0 0
  line L31 (63.547, 61.8836) -> (63.8931, 61.5253)
  arc A63 (63.8889, 60.8262) -> (63.8931, 61.5253) centre (63.5335, 61.1779) ccw
  arc A64 (63.8889, 60.8262) -> (63.0828, 59.9679) centre (79.882, 45) ccw
  arc A65 (62.3854, 59.9198) -> (63.0828, 59.9679) centre (62.7095, 60.3005) ccw
  line L32 (62.3854, 59.9198) -> (62.0061, 60.2427)
  spline S32 degree 5 poles (62.0061, 60.2427) (61.9982, 60.2493) (61.9824, 60.2625) (61.9582, 60.2816) (61.9251, 60.3059) (61.8825, 60.3347) (61.839, 60.3624) (61.795, 60.3894) (61.7507, 60.4161) (61.7061, 60.4424) (61.6614, 60.4685) (61.6164, 60.4943) (61.571, 60.5195) (61.5252, 60.5442) (61.479, 60.5684) (61.4325, 60.592) (61.3856, 60.6152) (61.3384, 60.638) (61.2911, 60.6605) (61.2435, 60.6826) (61.1957, 60.7045) (61.1476, 60.726) (61.0993, 60.7472) (61.0508, 60.768) (61.0021, 60.7885) (60.9531, 60.8086) (60.9039, 60.8284) (60.8545, 60.8479) (60.8049, 60.8671) (60.7551, 60.8859) (60.7051, 60.9045) (60.655, 60.9229) (60.6046, 60.9409) (60.5541, 60.9586) (60.5034, 60.976) (60.4525, 60.9931) (60.4015, 61.01) (60.3502, 61.0266) (60.2988, 61.0429) (60.2473, 61.0589) (60.1956, 61.0747) (60.1437, 61.0902) (60.0917, 61.1054) (60.0395, 61.1204) (59.9872, 61.1351) (59.9348, 61.1496) (59.8822, 61.1638) (59.8294, 61.1777) (59.7765, 61.1914) (59.7235, 61.2048) (59.6703, 61.218) (59.617, 61.2309) (59.5636, 61.2436) (59.51, 61.256) (59.4563, 61.2682) (59.4025, 61.2802) (59.3485, 61.2919) (59.2944, 61.3033) (59.2402, 61.3145) (59.1859, 61.3255) (59.1315, 61.3363) (59.0769, 61.3468) (59.0222, 61.357) (58.9675, 61.3671) (58.9125, 61.3769) (58.8575, 61.3864) (58.8024, 61.3957) (58.7472, 61.4048) (58.6918, 61.4137) (58.6364, 61.4224) (58.5808, 61.4308) (58.5363, 61.4373) (58.5028, 61.4421) (58.4805, 61.4453) (58.4694, 61.4468) knots 0 0 0 0 0 0 0.01428571 0.02857143 0.04285714 0.05714286 0.07142857 0.08571429 0.1 0.11428571 0.12857143 0.14285714 0.15714286 0.17142857 0.18571429 0.2 0.21428571 0.22857143 0.24285714 0.25714286 0.27142857 0.28571429 0.3 0.31428571 0.32857143 0.34285714 0.35714286 0.37142857 0.38571429 0.4 0.41428571 0.42857143 0.44285714 0.45714286 0.47142857 0.48571429 0.5 0.51428571 0.52857143 0.54285714 0.55714286 0.57142857 0.58571429 0.6 0.61428571 0.62857143 0.64285714 0.65714286 0.67142857 0.68571429 0.7 0.71428571 0.72857143 0.74285714 0.75714286 0.77142857 0.78571429 0.8 0.81428571 0.82857143 0.84285714 0.85714286 0.87142857 0.88571429 0.9 0.91428571 0.92857143 0.94285714 0.95714286 0.97142857 0.98571429 1 1 1 1 1 1
  arc A66 (58.4694, 61.4468) -> (57.6233, 60.2823) centre (79.882, 45) ccw
  spline S33 degree 5 poles (57.6233, 60.2823) (57.6282, 60.2722) (57.6381, 60.2519) (57.653, 60.2216) (57.673, 60.1813) (57.6982, 60.131) (57.7235, 60.0809) (57.7491, 60.0311) (57.7748, 59.9813) (57.8007, 59.9318) (57.8268, 59.8824) (57.8531, 59.8332) (57.8795, 59.7842) (57.9062, 59.7354) (57.933, 59.6868) (57.9601, 59.6383) (57.9873, 59.59) (58.0147, 59.5419) (58.0423, 59.4941) (58.0701, 59.4464) (58.0981, 59.3989) (58.1263, 59.3516) (58.1547, 59.3045) (58.1833, 59.2575) (58.212, 59.2108) (58.241, 59.1644) (58.2702, 59.1181) (58.2995, 59.072) (58.3291, 59.0261) (58.3588, 58.9805) (58.3888, 58.935) (58.4189, 58.8898) (58.4493, 58.8448) (58.4799, 58.8001) (58.5106, 58.7555) (58.5416, 58.7112) (58.5728, 58.6672) (58.6042, 58.6233) (58.6358, 58.5798) (58.6676, 58.5364) (58.6996, 58.4933) (58.7318, 58.4505) (58.7643, 58.4079) (58.797, 58.3656) (58.8299, 58.3235) (58.863, 58.2818) (58.8964, 58.2402) (58.93, 58.199) (58.9638, 58.158) (58.9978, 58.1174) (59.0321, 58.077) (59.0666, 58.0369) (59.1014, 57.9972) (59.1364, 57.9579) (59.1718, 57.9188) (59.2073, 57.8801) (59.2431, 57.8417) (59.2791, 57.8036) (59.3154, 57.7658) (59.3519, 57.7283) (59.3888, 57.6914) (59.426, 57.6549) (59.4637, 57.619) (59.5017, 57.5837) (59.5401, 57.5488) (59.5788, 57.5143) (59.6176, 57.4801) (59.6566, 57.4462) (59.6959, 57.4126) (59.7357, 57.3798) (59.7763, 57.3482) (59.8096, 57.3243) (59.8353, 57.3072) (59.8526, 57.2962) (59.8614, 57.2908) knots -1 -1 -1 -1 -1 -1 -0.98571429 -0.97142857 -0.95714286 -0.94285714 -0.92857143 -0.91428571 -0.9 -0.88571429 -0.87142857 -0.85714286 -0.84285714 -0.82857143 -0.81428571 -0.8 -0.78571429 -0.77142857 -0.75714286 -0.74285714 -0.72857143 -0.71428571 -0.7 -0.68571429 -0.67142857 -0.65714286 -0.64285714 -0.62857143 -0.61428571 -0.6 -0.58571429 -0.57142857 -0.55714286 -0.54285714 -0.52857143 -0.51428571 -0.5 -0.48571429 -0.47142857 -0.45714286 -0.44285714 -0.42857143 -0.41428571 -0.4 -0.38571429 -0.37142857 -0.35714286 -0.34285714 -0.32857143 -0.31428571 -0.3 -0.28571429 -0.27142857 -0.25714286 -0.24285714 -0.22857143 -0.21428571 -0.2 -0.18571429 -0.17142857 -0.15714286 -0.14285714 -0.12857143 -0.11428571 -0.1 -0.08571429 -0.07142857 -0.05714286 -0.04285714 -0.02857143 -0.01428571 0 0 0 0 0 0
  line L33 (59.8614, 57.2908) -> (60.2857, 57.0298)
  arc A67 (60.4555, 56.3517) -> (60.2857, 57.0298) centre (60.0238, 56.6039) ccw
  arc A68 (60.4555, 56.3517) -> (59.8882, 55.3198) centre (79.882, 45) ccw
  arc A69 (59.2247, 55.0998) -> (59.8882, 55.3198) centre (59.4439, 55.5491) ccw
  line L34 (59.2247, 55.0998) -> (58.777, 55.3182)
  spline S34 degree 5 poles (58.777, 55.3182) (58.7677, 55.3227) (58.7491, 55.3315) (58.721, 55.344) (58.6829, 55.3593) (58.6344, 55.3767) (58.5854, 55.3927) (58.5361, 55.4079) (58.4865, 55.4227) (58.4368, 55.4371) (58.387, 55.4513) (58.337, 55.465) (58.2867, 55.4782) (58.2362, 55.4907) (58.1855, 55.5026) (58.1345, 55.514) (58.0834, 55.5248) (58.032, 55.5351) (57.9805, 55.5451) (57.9289, 55.5547) (57.8772, 55.564) (57.8253, 55.5729) (57.7733, 55.5814) (57.7211, 55.5895) (57.6688, 55.5972) (57.6163, 55.6045) (57.5638, 55.6114) (57.5111, 55.618) (57.4582, 55.6243) (57.4053, 55.6302) (57.3523, 55.6358) (57.2992, 55.641) (57.2459, 55.646) (57.1926, 55.6506) (57.1391, 55.6548) (57.0856, 55.6588) (57.0319, 55.6624) (56.9782, 55.6657) (56.9244, 55.6687) (56.8705, 55.6715) (56.8165, 55.6739) (56.7624, 55.676) (56.7082, 55.6778) (56.654, 55.6793) (56.5996, 55.6806) (56.5452, 55.6815) (56.4907, 55.6822) (56.4362, 55.6826) (56.3815, 55.6827) (56.3268, 55.6825) (56.272, 55.682) (56.2172, 55.6813) (56.1623, 55.6803) (56.1073, 55.679) (56.0523, 55.6775) (55.9972, 55.6756) (55.942, 55.6735) (55.8868, 55.6712) (55.8315, 55.6686) (55.7761, 55.6657) (55.7207, 55.6626) (55.6653, 55.6592) (55.6098, 55.6555) (55.5542, 55.6516) (55.4986, 55.6474) (55.4429, 55.643) (55.3872, 55.6384) (55.3314, 55.6334) (55.2756, 55.6283) (55.2198, 55.6228) (55.1639, 55.6172) (55.1191, 55.6124) (55.0855, 55.6088) (55.0631, 55.6063) (55.0519, 55.605) knots 0 0 0 0 0 0 0.01428571 0.02857143 0.04285714 0.05714286 0.07142857 0.08571429 0.1 0.11428571 0.12857143 0.14285714 0.15714286 0.17142857 0.18571429 0.2 0.21428571 0.22857143 0.24285714 0.25714286 0.27142857 0.28571429 0.3 0.31428571 0.32857143 0.34285714 0.35714286 0.37142857 0.38571429 0.4 0.41428571 0.42857143 0.44285714 0.45714286 0.47142857 0.48571429 0.5 0.51428571 0.52857143 0.54285714 0.55714286 0.57142857 0.58571429 0.6 0.61428571 0.62857143 0.64285714 0.65714286 0.67142857 0.68571429 0.7 0.71428571 0.72857143 0.74285714 0.75714286 0.77142857 0.78571429 0.8 0.81428571 0.82857143 0.84285714 0.85714286 0.87142857 0.88571429 0.9 0.91428571 0.92857143 0.94285714 0.95714286 0.97142857 0.98571429 1 1 1 1 1 1
  arc A70 (55.0519, 55.605) -> (54.522, 54.2666) centre (79.882, 45) ccw
  spline S35 degree 5 poles (54.522, 54.2666) (54.5293, 54.2581) (54.544, 54.2409) (54.5659, 54.2152) (54.5953, 54.1811) (54.6322, 54.1387) (54.6692, 54.0966) (54.7063, 54.0546) (54.7436, 54.0128) (54.781, 53.9713) (54.8186, 53.93) (54.8563, 53.8888) (54.8941, 53.848) (54.9321, 53.8073) (54.9702, 53.7669) (55.0084, 53.7266) (55.0468, 53.6867) (55.0853, 53.6469) (55.1239, 53.6074) (55.1627, 53.5681) (55.2017, 53.5291) (55.2407, 53.4903) (55.2799, 53.4517) (55.3193, 53.4134) (55.3587, 53.3753) (55.3984, 53.3374) (55.4381, 53.2999) (55.478, 53.2625) (55.518, 53.2255) (55.5582, 53.1886) (55.5985, 53.1521) (55.639, 53.1158) (55.6796, 53.0798) (55.7203, 53.044) (55.7612, 53.0085) (55.8022, 52.9733) (55.8434, 52.9384) (55.8847, 52.9038) (55.9261, 52.8694) (55.9677, 52.8353) (56.0094, 52.8015) (56.0513, 52.7681) (56.0934, 52.7349) (56.1355, 52.702) (56.1779, 52.6695) (56.2203, 52.6373) (56.263, 52.6054) (56.3057, 52.5738) (56.3487, 52.5425) (56.3917, 52.5116) (56.435, 52.481) (56.4784, 52.4508) (56.522, 52.421) (56.5657, 52.3916) (56.6096, 52.3625) (56.6537, 52.3339) (56.6979, 52.3056) (56.7423, 52.2776) (56.7868, 52.25) (56.8315, 52.2228) (56.8764, 52.1962) (56.9215, 52.1701) (56.9669, 52.1447) (57.0126, 52.12) (57.0584, 52.0957) (57.1044, 52.0719) (57.1506, 52.0485) (57.1968, 52.0253) (57.2432, 52.0026) (57.2899, 51.9807) (57.337, 51.9602) (57.3753, 51.9453) (57.4044, 51.9351) (57.424, 51.9288) (57.4338, 51.9257) knots -1 -1 -1 -1 -1 -1 -0.98571429 -0.97142857 -0.95714286 -0.94285714 -0.92857143 -0.91428571 -0.9 -0.88571429 -0.87142857 -0.85714286 -0.84285714 -0.82857143 -0.81428571 -0.8 -0.78571429 -0.77142857 -0.75714286 -0.74285714 -0.72857143 -0.71428571 -0.7 -0.68571429 -0.67142857 -0.65714286 -0.64285714 -0.62857143 -0.61428571 -0.6 -0.58571429 -0.57142857 -0.55714286 -0.54285714 -0.52857143 -0.51428571 -0.5 -0.48571429 -0.47142857 -0.45714286 -0.44285714 -0.42857143 -0.41428571 -0.4 -0.38571429 -0.37142857 -0.35714286 -0.34285714 -0.32857143 -0.31428571 -0.3 -0.28571429 -0.27142857 -0.25714286 -0.24285714 -0.22857143 -0.21428571 -0.2 -0.18571429 -0.17142857 -0.15714286 -0.14285714 -0.12857143 -0.11428571 -0.1 -0.08571429 -0.07142857 -0.05714286 -0.04285714 -0.02857143 -0.01428571 0 0 0 0 0 0
  line L35 (57.4338, 51.9257) -> (57.9097, 51.7785)
  arc A71 (58.2428, 51.1639) -> (57.9097, 51.7785) centre (57.7619, 51.3008) ccw
  arc A72 (58.2428, 51.1639) -> (57.9499, 50.0233) centre (79.882, 45) ccw
  arc A73 (57.3619, 49.6452) -> (57.9499, 50.0233) centre (57.4626, 50.135) ccw
  line L36 (57.3619, 49.6452) -> (56.874, 49.7455)
  spline S36 degree 5 poles (56.874, 49.7455) (56.8639, 49.7475) (56.8437, 49.7514) (56.8133, 49.7565) (56.7726, 49.7619) (56.7214, 49.7666) (56.6699, 49.7699) (56.6183, 49.7724) (56.5667, 49.7744) (56.5149, 49.776) (56.4632, 49.7773) (56.4113, 49.7782) (56.3594, 49.7785) (56.3073, 49.7781) (56.2552, 49.777) (56.2031, 49.7753) (56.1508, 49.773) (56.0985, 49.7703) (56.0461, 49.7671) (55.9938, 49.7636) (55.9413, 49.7597) (55.8889, 49.7554) (55.8364, 49.7507) (55.7838, 49.7456) (55.7312, 49.7401) (55.6786, 49.7341) (55.626, 49.7277) (55.5733, 49.721) (55.5206, 49.7139) (55.4679, 49.7065) (55.4151, 49.6987) (55.3623, 49.6906) (55.3095, 49.6821) (55.2567, 49.6733) (55.2039, 49.6642) (55.151, 49.6547) (55.0982, 49.6448) (55.0453, 49.6347) (54.9924, 49.6242) (54.9395, 49.6135) (54.8866, 49.6024) (54.8337, 49.591) (54.7808, 49.5793) (54.7279, 49.5672) (54.6749, 49.5549) (54.622, 49.5423) (54.569, 49.5294) (54.5161, 49.5162) (54.4632, 49.5027) (54.4102, 49.4889) (54.3573, 49.4749) (54.3043, 49.4605) (54.2514, 49.4459) (54.1985, 49.431) (54.1455, 49.4158) (54.0926, 49.4003) (54.0397, 49.3846) (53.9868, 49.3686) (53.9339, 49.3523) (53.881, 49.3357) (53.8281, 49.3189) (53.7753, 49.3018) (53.7224, 49.2845) (53.6696, 49.2669) (53.6167, 49.249) (53.5639, 49.2309) (53.5111, 49.2125) (53.4583, 49.1939) (53.4055, 49.175) (53.3528, 49.1559) (53.3001, 49.1365) (53.2579, 49.1207) (53.2263, 49.1088) (53.2052, 49.1009) (53.1946, 49.0969) knots 0 0 0 0 0 0 0.01428571 0.02857143 0.04285714 0.05714286 0.07142857 0.08571429 0.1 0.11428571 0.12857143 0.14285714 0.15714286 0.17142857 0.18571429 0.2 0.21428571 0.22857143 0.24285714 0.25714286 0.27142857 0.28571429 0.3 0.31428571 0.32857143 0.34285714 0.35714286 0.37142857 0.38571429 0.4 0.41428571 0.42857143 0.44285714 0.45714286 0.47142857 0.48571429 0.5 0.51428571 0.52857143 0.54285714 0.55714286 0.57142857 0.58571429 0.6 0.61428571 0.62857143 0.64285714 0.65714286 0.67142857 0.68571429 0.7 0.71428571 0.72857143 0.74285714 0.75714286 0.77142857 0.78571429 0.8 0.81428571 0.82857143 0.84285714 0.85714286 0.87142857 0.88571429 0.9 0.91428571 0.92857143 0.94285714 0.95714286 0.97142857 0.98571429 1 1 1 1 1 1
  arc A74 (53.1946, 49.0969) -> (53.0142, 47.6687) centre (79.882, 45) ccw